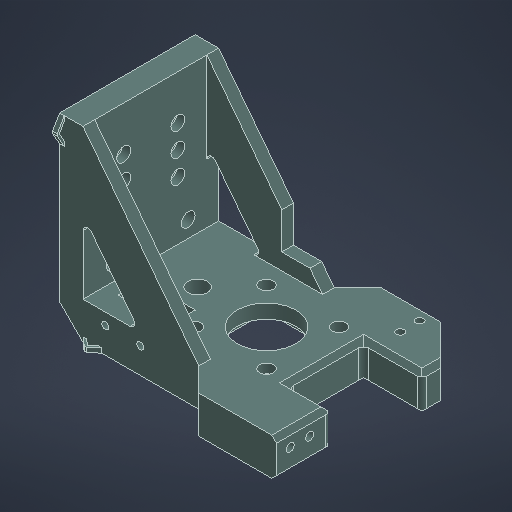
# Autodesk Inventor part: HolderV2
Saved by Autodesk Inventor 2025.1 (Build 291241000, 241)
## iProperties
Created: 2025-03-02
Part Number: HolderV2
Material: Generic
Document SubType Name: Modeling
Designer: 13156
Density: 1 g/cm^3
Appearance: Default
Author: 13156
## iProperties of the stored document HolderV2_3DPrint.ipt
Created: 2025-03-03
Part Number: HolderV2_3DPrint
Material: Generic
Document SubType Name: Modeling
Designer: jerem
Density: 1 g/cm^3
Appearance: Default
Author: jerem
Autodesk Inventor part; units mm, degrees
ref_plane "YZ Plane" through (0, 0, 0) normal (1, 0, 0) x (0, 1, 0)
ref_plane "XZ Plane" through (0, 0, 0) normal (0, 1, 0) x (-1, 0, 0)
ref_plane "XY Plane" through (0, 0, 0) normal (0, 0, 1) x (1, 0, 0)
sketch "Sketch1" plane through (0, 0, 0) normal (0, 1, 0) x (-1, 0, 0)
  line L0 (55, 39) -> (-55, 39)
  line L1 (-55, 39) -> (-55, -39)
  line L2 (-55, -39) -> (55, -39)
  line L3 (55, -39) -> (55, 39)
  line L4 (0, 0) -> (-9, 0) construction
  line L5 (0, 0) -> (0, -15.5) construction
  circle A0 centre (-4.5, 0) radius 12.5
  line L6 (17, 21.5) -> (-26, 21.5)
  line L7 (-26, 21.5) -> (-26, -21.5)
  line L8 (-26, -21.5) -> (17, -21.5)
  line L9 (-55, 16) -> (-30, 16)
  line L10 (-30, 16) -> (-30, -16)
  line L11 (-30, -16) -> (-55, -16)
  line L12 (-55, -16) -> (-55, 16)
  circle A1 centre (-35, -26.7) radius 1.7
  circle A2 centre (-35, -35) radius 1.7
  line L13 (17, 21.5) -> (17, -21.5)
  circle A3 centre (25, 0) radius 4.2
  line L14 (-55, 39) -> (-47.75, 39)
  line L15 (-47.75, 39) -> (-47.75, 16)
  line L16 (-47.75, 16) -> (-55, 16)
  line L17 (-55, 16) -> (-55, 39)
  line L18 (-4.5, 0) -> (55, 0) construction
  circle A4 centre (11, 15.5) radius 1.7
  circle A5 centre (11, -15.5) radius 1.7
  circle A6 centre (-20, -15.5) radius 1.7
  circle A7 centre (-20, 15.5) radius 1.7
  line L19 (-20, 15.5) -> (11, 15.5) construction
  line L20 (-20, 15.5) -> (-20, -15.5) construction
  line L21 (-20, -15.5) -> (11, -15.5) construction
  line L22 (11, -15.5) -> (11, 15.5) construction
  line L23 (-35, -26.7) -> (-35, -54.4551) construction
  line L24 (55, 39) -> (45, 39)
  line L25 (45, 39) -> (45, -39)
  line L26 (45, -39) -> (55, -39)
  line L27 (55, -39) -> (55, 39)
  line L28 (55, 39) -> (-4.5, 39)
  line L29 (-4.5, 39) -> (-4.5, 29)
  line L30 (-4.5, 29) -> (55, 29)
  line L31 (55, 29) -> (55, 39)
  line L32 (55, -39) -> (-4.5, -39)
  line L33 (-4.5, -39) -> (-4.5, -29)
  line L34 (-4.5, -29) -> (55, -29)
  line L35 (55, -29) -> (55, -39)
  line L36 (-4.5, 0) -> (-4.5, 17.2) construction
  circle A8 centre (-20, 15.5) radius 3
  circle A9 centre (11, 15.5) radius 3
  circle A10 centre (11, -15.5) radius 3
  circle A11 centre (-20, -15.5) radius 3
  point P0 (-55, -16)
  point P1 (-4.5, 39)
  point P2 (-4.5, -39)
  point P3 (55, 0)
  dimension "d0" = 78
  dimension "d1" = 110
  dimension "d3" = 25
  dimension "d5" = 25
  dimension "d6" = 43
  dimension "d7" = 21.5
  dimension "d8" = 8.4
  dimension "d9" = 30
  dimension "d11" = 3.4
  dimension "d12" = 6
  dimension "d13" = 6
  dimension "d14" = 6
  dimension "d15" = 6
  dimension "d16" = 3.4
  dimension "d17" = 4
  dimension "d18" = 8.3
  dimension "d19" = 5
  dimension "d20" = 5
  dimension "d21" = 10
  dimension "d51" = 10
  dimension "d108" = 7.25
  dimension "d109" = 32
  dimension "d110" = 59.5
  dimension "d150" = 6
  constraints: 77 end point, 13 parallel, 12 centre point, 11 horizontal, 11 perpendicular, 7 equal radius, 5 coincident, 5 point on line, 3 midpoint, 3 vertical, 2 collinear, 5 other
  measures "d0" distance of L2.end L0.start
  measures "d1" distance of L1.end L2.end
  measures "d3" distance between parallel lines of L1 L10
  measures "d5" diameter of A0
  measures "d6" distance of L6.start L8.end
  measures "d7" distance from line of L13 L18.start
  measures "d8" diameter of A3
  measures "d9" distance of L18.end A3.centre
  measures "d11" diameter of A4
  measures "d12" distance from line of L6 L19.start
  measures "d13" distance from line of L7 L19.start
  measures "d14" distance from line of L13 L21.end
  measures "d15" distance between parallel lines of L8 L21
  measures "d16" diameter of A1
  measures "d17" distance from line of L2 A2.centre
  measures "d18" distance of L23.start A2.centre
  measures "d19" distance from line of L10 L23.start
  measures "d20" distance from line of L10 A2.centre
  measures "d21" distance between parallel lines of L27 L25
  measures "d51" distance between parallel lines of L32 L34
  measures "d108" distance of L0.end L14.end
  measures "d109" distance of L11.end L9.start
  measures "d110" distance of point (55, 0) L18.start
  measures "d150" diameter of A8
extrude "Extrusion1" add sketch "Sketch1" along normal blind 16 contours L3 L30 L25 L0 | L25 L30 L29 L0 | L3 L34 L25 L30 | L29 L30 L25 L34 L33 L2 L1 L11 L10 L9 L15 L0 | L3 L2 L25 L34 | L25 L2 L33 L34 | L13 L8 L7 L6 | A8 | A9 | A10 | A11
extrude "Extrusion21" cut sketch "Sketch1" against normal blind 4 from surface at 16 contours A8 | A9 | A10 | A11
extrude "Extrusion2" add sketch "Sketch1" along normal blind 80 contours L3 L30 L25 L0 | L3 L34 L25 L30 | L3 L2 L25 L34
ref_plane "Work Plane1" through (0, 10, 0) normal (0, -1, 0) x (1, 0, 0)
extrude "Extrusion3" cut sketch "Sketch1" along normal up to surface (10 mm away) contours A0 | L13 L8 L7 L6 | A4 | A5 | A6 | A7 | A8 | A9 | A10 | A11
sketch "Sketch2" plane through (47.75, 0, 39) normal (1, 0, 0) x (0, 0, -1)
  circle A0 centre (5.925, 9.5) radius 1.7
  circle A1 centre (14.225, 9.5) radius 1.7
  line L0 (0, 16) -> (23, 16) projected
  line L1 (5.925, 9.5) -> (23.5795, 9.5) construction
  line L2 (0, 0) -> (0, 16) construction
  point P0 (39, 0)
  point P1 (0, 8)
  dimension "d29" = 3.4
  dimension "d30" = 6.5
  dimension "d31" = 8.3
  dimension "d32" = 5.925
  constraints: 2 centre point, 2 end point, 1 equal radius, 1 horizontal, 1 midpoint, 1 point on line
  measures "d29" diameter of A0
  measures "d30" distance from line of L0 L1.start
  measures "d31" distance of L1.start A1.centre
  measures "d32" horizontal distance of point (0, 8) L1.start
extrude "Extrusion4" cut sketch "Sketch2" against normal blind 8
sketch "Sketch3" plane through (-45, 16, -39) normal (1, 0, 0) x (0, 0, -1)
  circle A0 centre (-55, 7) radius 2.95
  circle A1 centre (-23, 7) radius 2.95
  circle A2 centre (-50.6, 45) radius 1.5
  circle A3 centre (-27.4, 45) radius 1.5
  circle A4 centre (-50.6, 35) radius 1.5
  circle A5 centre (-27.4, 35) radius 1.5
  circle A6 centre (-50.6, 25) radius 1.5
  circle A7 centre (-27.4, 25) radius 1.5
  line L0 (-111.9062, 0) -> (57.702, 0) construction
  line L1 (-39, -16) -> (-39, 45) construction
  line L2 (-50.6, 82.5983) -> (-50.6, 7.4017) construction
  line L3 (-27.4, 83) -> (-27.4, 7) construction
  line L4 (-23, 0) -> (0, 0) construction
  line L5 (-23, 7) -> (-55, 7) construction
  line L6 (-27.4, 45) -> (-50.6, 45) construction
  line L7 (-27.4, 35) -> (-50.6, 35) construction
  line L8 (-27.4, 25) -> (-50.6, 25) construction
  line L9 (-27.4, 15) -> (-50.6, 15) construction
  circle A8 centre (-27.4, 45) radius 3
  circle A9 centre (-27.4, 35) radius 3
  circle A10 centre (-27.4, 25) radius 3
  circle A11 centre (-50.6, 25) radius 3
  circle A12 centre (-50.6, 35) radius 3
  circle A13 centre (-50.6, 45) radius 3
  line L10 (-50.95, 9.3383) -> (-50.95, 4.6617)
  line L11 (-50.95, 4.6617) -> (-55, 2.3235)
  line L12 (-55, 2.3235) -> (-59.05, 4.6617)
  line L13 (-59.05, 4.6617) -> (-59.05, 9.3383)
  line L14 (-59.05, 9.3383) -> (-55, 11.6765)
  line L15 (-55, 11.6765) -> (-50.95, 9.3383)
  line L16 (-18.95, 4.6617) -> (-23, 2.3235)
  line L17 (-23, 2.3235) -> (-27.05, 4.6617)
  line L18 (-27.05, 4.6617) -> (-27.05, 9.3383)
  line L19 (-27.05, 9.3383) -> (-23, 11.6765)
  line L20 (-23, 11.6765) -> (-18.95, 9.3383)
  line L21 (-18.95, 9.3383) -> (-18.95, 4.6617)
  line L22 (-55, 0) -> (-23, 0) projected
  point P0 (-27.1021, 0)
  dimension "d35" = 5.9
  dimension "d36" = 0
  dimension "d37" = 7
  dimension "d38" = 16
  dimension "d39" = 23.2
  dimension "d41" = 10
  dimension "d42" = 45
  dimension "d43" = 10
  dimension "d44" = 10
  dimension "d45" = 6
  dimension "d118" = 3
  dimension "d121" = 8.1
  constraints: 46 end point, 14 centre point, 11 equal radius, 8 coincident, 7 point on line, 6 horizontal, 6 midpoint, 5 vertical, 2 perpendicular, 1 equal length, 1 symmetric about line, 27 other
  measures "d35" diameter of A0
  measures "d36" distance between parallel lines of L4 L0
  measures "d37" distance from line of L5.start L4
  measures "d38" distance from line of L1 L5.start
  measures "d39" distance of L6.end L6.start
  measures "d41" distance of L7.start L6.start
  measures "d42" vertical distance of point (-27.102, 0) L6.start
  measures "d43" distance of L8.start L7.start
  measures "d44" distance of L8.start L9.start
  measures "d45" diameter of A13
  measures "d118" diameter of A2
  measures "d121" distance between parallel lines of L10 L13
extrude "Extrusion5" cut sketch "Sketch3" against normal blind 22.2875 contours A0 | A1 | A2 | A3 | A4 | A5 | A6 | A7
extrude "Extrusion6" cut sketch "Sketch3" against normal blind 3.5 contours A2 | A3 | A4 | A5 | A6 | A7 | A8 | A9 | A10 | A11 | A12 | A13
extrude "Extrusion7" cut sketch "Sketch1" along normal blind 90 contours L3 L30 L25 L0 | L25 L30 L29 L0 | L3 L2 L25 L34 | L25 L2 L33 L34
sketch "Sketch4" plane through (-55, 0, 29) normal (0, 0, 1) x (1, 0, 0)
  point P0 (55, 0)
chamfer "Chamfer1" distance 10 angle 45 2 edges at (4.5, 8, -39) (4.5, 8, 39)
sketch "Sketch5" plane through (-55, 80, 29) normal (0, 0, 1) x (1, 0, 0)
  line L0 (10, -64) -> (10, 0) projected
  line L1 (10, 0) -> (59.5, -64)
  line L2 (59.5, -64) -> (34.216, -64)
  line L3 (10, -64) -> (59.5, -64) projected
  line L4 (34.216, -64) -> (10, -32.6905)
  line L5 (10, -32.6905) -> (10, 0)
  line L6 (10, 0) -> (10, -32.6905)
  line L7 (42, -41.3737) -> (54.0859, -41.3737)
  line L8 (54.0859, -41.3737) -> (54.0859, -57)
  line L9 (54.0859, -57) -> (42, -57)
  line L10 (42, -57) -> (42, -41.3737)
  point P0 (55, -80)
  point P1 (10, -32.6905)
  point P2 (48.043, -57)
  point P3 (42, -49.1869)
  dimension "d57" = 20
  dimension "d97" = 7
  dimension "d99" = 17.5
  constraints: 18 end point, 3 parallel, 3 point on line, 2 midpoint, 2 perpendicular, 1 collinear, 1 horizontal
  measures "d57" distance between parallel lines of L1 L4
  measures "d97" distance from line of L2 point (48.043, -57)
  measures "d99" horizontal distance of L1.end point (42, -49.187)
ref_plane "Work Plane2" through (-45, 80, 0) normal (0, 0, -1) x (-1, 0, 0)
chamfer "Chamfer3" distance 2 angle 45 10 edges at (30, 16, 0) (38.875, 16, 16) (42.5, 16, -16) (42.5, 0, -16) (30, 0, 0) (38.875, 0, 16) (47.75, 0, 27.5) (47.75, 16, 27.5) (55, 16, -27.5) (55, 0, -27.5)
fillet "Fillet3" radius 2 4 edges at (30, 8, 16) (30, 8, -16) (47.75, 8, 16) (55, 8, -16) curvature continuous yes
extrude "Extrusion13" add sketch "Sketch5" against normal blind 5 contours L0 L1 L10 L9 L2 L4 | L1 L9 L10
ref_plane "Work Plane4" through (-45, 80, 0) normal (0, 0, -1) x (-1, 0, 0)
mirror "Mirror2" about plane through (-45, 80, 0) normal (0, 0, -1) of "Extrusion13"
extrude "Extrusion14" cut sketch "Sketch5" along normal up to surface (5 mm away) from surface at -58 contours L1 L9 L10
sketch "Sketch6" plane through (14.5, 0, -39) normal (0, 0, -1) x (-1, 0, 0)
  circle A0 centre (-14.5, 11) radius 1.7
  line L0 (-40.5, 16) -> (0, 16) projected
  line L1 (-14.5, 33.6325) -> (-14.5, -16.3308) construction
  line L2 (-40.5, 0) -> (-40.5, 16) construction
  point P0 (14.5, 0)
  point P1 (-38.5, 16)
  point P2 (-40.5, 2)
  point P3 (-40.5, 14)
  dimension "d102" = 3.4
  dimension "d103" = 5
  dimension "d105" = 26
  constraints: 2 end point, 1 centre point, 1 point on line, 1 vertical
  measures "d102" diameter of A0
  measures "d103" distance from line of L0 A0.centre
  measures "d105" distance between parallel lines of L2 L1
extrude "Extrusion15" cut sketch "Sketch6" against normal blind 8
chamfer "Chamfer7" distance 10 angle 45 1 edges at (-55, 0, 0)
fillet "Fillet8" radius 2 4 edges at (-20.784, 16, -26.5) (-45, 47.3095, -26.5) (-20.784, 16, 26.5) (-45, 47.3095, 26.5)
extrude "Extrusion16" cut sketch "Sketch3" along normal blind 4 from surface at -10 contours A0 | L10 L11 L12 L13 L14 L15 | L16 L17 L18 L19 L20 L21
sketch "Sketch7" plane through (0, 16, 0) normal (0, 1, 0) x (1, 0, 0)
  line L0 (-45, -24) -> (4.5, -24) construction
  line L1 (-45, -24) -> (-45, 24) projected
  line L2 (-39, -20) -> (-39, -9)
  line L3 (-39, -9) -> (-17, -9)
  line L4 (-17, -9) -> (-17, -20)
  line L5 (-17, -20) -> (-39, -20)
  point P0 (0, 0)
  dimension "d124" = 22
  dimension "d125" = 6
  dimension "d148" = 11
  dimension "d149" = 4
  constraints: 8 end point, 2 perpendicular, 1 horizontal, 1 vertical
  measures "d124" distance of L2.end L3.end
  measures "d125" distance between parallel lines of L1 L2
  measures "d148" distance between parallel lines of L5 L3
  measures "d149" distance between parallel lines of L0 L5
extrude "Extrusion17" cut sketch "Sketch7" against normal through all
sketch "Sketch8" plane through (-55, 80, 29) normal (0, 0, 1) x (1, 0, 0)
  line L0 (16, -64) -> (38, -64) projected
  circle A0 centre (19.5, -69) radius 1.5
  circle A1 centre (34.5, -69) radius 1.5
  line L1 (19.5, -69) -> (34.5, -69) construction
  line L2 (27, -69) -> (27, -64) construction
  line L3 (10, -64) -> (30.1407, -64) construction
  point P0 (55, -80)
  dimension "d128" = 3
  dimension "d129" = 15
  dimension "d132" = 5
  constraints: 4 end point, 2 centre point, 2 midpoint, 1 equal radius, 1 horizontal, 1 perpendicular
  measures "d128" diameter of A0
  measures "d129" distance of L1.start L1.end
  measures "d132" distance of L2.start L2.end
extrude "Extrusion18" cut sketch "Sketch8" against normal blind 10
sketch "Sketch9" plane through (-55, 80, -29) normal (-1, 0, 0) x (0, 0, 1)
  line L0 (40.95, -54.6617) -> (45, -52.3235) projected
  line L1 (45, -52.3235) -> (49.05, -54.6617) projected
  line L2 (49.05, -54.6617) -> (49.05, -59.3383) projected
  line L3 (49.05, -59.3383) -> (45, -61.6765) projected
  line L4 (45, -61.6765) -> (40.95, -59.3383) projected
  line L5 (40.95, -59.3383) -> (40.95, -54.6617) projected
  line L6 (8.95, -59.3383) -> (8.95, -54.6617) projected
  line L7 (8.95, -54.6617) -> (13, -52.3235) projected
  line L8 (13, -52.3235) -> (17.05, -54.6617) projected
  line L9 (17.05, -54.6617) -> (17.05, -59.3383) projected
  line L10 (17.05, -59.3383) -> (13, -61.6765) projected
  line L11 (13, -61.6765) -> (8.95, -59.3383) projected
  line L12 (58, -70) -> (0, -70) projected
  line L13 (58, -70) -> (58, 0) projected
  line L14 (0, 0) -> (58, 0) projected
  line L15 (0, 0) -> (0, -70) projected
  circle A0 centre (40.6, -19) radius 1.5 projected
  circle A1 centre (17.4, -29) radius 1.5 projected
  circle A2 centre (17.4, -19) radius 1.5 projected
  circle A3 centre (40.6, -29) radius 1.5 projected
  circle A4 centre (17.4, -39) radius 1.5 projected
  circle A5 centre (40.6, -39) radius 1.5 projected
  line L16 (29, 0) -> (29, -70) construction
  line L17 (0, 0) -> (-3, -5.1962)
  line L18 (-3, -5.1962) -> (-3, -6.1962)
  line L19 (-3, -6.1962) -> (0, -11.3923)
  line L20 (0.866, -0.5) -> (-2, -5.4641)
  line L21 (-2, -5.4641) -> (-2, -5.9282)
  line L22 (-2, -5.9282) -> (0.866, -10.8923)
  line L23 (58, 0) -> (61, -5.1962)
  line L24 (61, -5.1962) -> (61, -6.1962)
  line L25 (61, -6.1962) -> (58, -11.3923)
  line L26 (57.134, -0.5) -> (60, -5.4641)
  line L27 (60, -5.4641) -> (60, -5.9282)
  line L28 (60, -5.9282) -> (57.134, -10.8923)
  point P0 (29, -80)
  point P1 (-3, -5.6962)
  point P2 (58, -2)
  point P3 (58, -9.3923)
  point P4 (58, -11.3923)
  point P5 (0, -9.3923)
  point P6 (0, -2)
  dimension "d133" = 30
  dimension "d134" = 3
  dimension "d135" = 1
  dimension "d136" = 1
  constraints: 26 end point, 7 symmetric about line, 3 midpoint, 1 equal length, 1 parallel, 1 point on line, 2 other
  measures "d133" angle of L15 L19
  measures "d134" distance from line of L15 point (-3, -5.696)
  measures "d135" distance of L17.end L18.end
  measures "d136" distance between parallel lines of L17 L20
extrude "Extrusion19" add sketch "Sketch9" against normal blind 2 contours L13 L28 L27 L26 L23 L24 L25 | L19 L18 L17 L15 L20 L21 L22
sketch "Sketch10" plane through (0, 0, 0) normal (0, -1, 0) x (1, 0, 0)
  line L0 (-45, 29) -> (-41.5, 32)
  line L1 (-41.5, 32) -> (-40.5, 32)
  line L2 (-40.5, 32) -> (-37, 29)
  line L3 (-43.9173, 28.611) -> (-41.1301, 31)
  line L4 (-41.1301, 31) -> (-40.8699, 31)
  line L5 (-40.8699, 31) -> (-37.8258, 28.3908)
  line L6 (-45, 29) -> (-37, 29)
  point P0 (0, 0)
  point P1 (-43.4634, 29)
  point P2 (-38.5366, 29)
  dimension "d142" = 1
  dimension "d143" = 3
  dimension "d144" = 1
  dimension "d145" = 8
  constraints: 14 end point, 2 horizontal, 1 equal length, 2 other
  measures "d142" distance of L0.end L1.end
  measures "d143" distance from line of L0.start L1
  measures "d144" distance between parallel lines of L0 L3
  measures "d145" distance of L0.start L2.end
extrude "Extrusion20" add sketch "Sketch10" against normal blind 2 contours L0 L1 L2 L6 L5 L4 L3
chamfer "Chamfer6" distance 15 angle 45 1 edges at (55, 8, -39)
equation "\"d14\" = d13"
equation "\"d15\" = d13"
equation "\"d20\" = d19"
body "Solid1"
